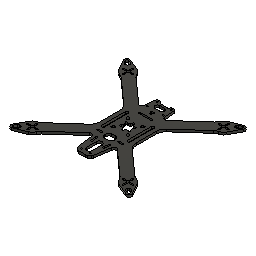
5inch test frame (Autodesk Fusion 360 design; units mm, degrees)
part number: 2026-08-20-13-27-36-607
Autodesk Fusion 360 part; units mm, degrees
note: some values were not read from the file. Chosen so that the rebuilt part matches the saved one: which bodies a step acts on.
(part 1 of 3)
sketch "reference" plane through (0, 0, 0) normal (0, 0, 1) x (1, 0, 0)
  line L0 (100, -100) -> (-100, -100) construction
  line L1 (-100, -100) -> (-100, 100) construction
  line L2 (-100, 100) -> (100, 100) construction
  line L3 (100, 100) -> (100, -100) construction
  line L4 (100, -100) -> (-100, 100) construction
  line L5 (-100, -100) -> (100, 100) construction
  circle A0 centre (-100, 100) radius 67.31
  circle A1 centre (100, 100) radius 67.31
  circle A2 centre (-100, -100) radius 67.31
  circle A3 centre (100, -100) radius 67.31
  line L6 (-32.69, 100) -> (32.69, 100)
  dimension "d1" = 134.62
  dimension "d2" = 134.62
  dimension "d3" = 134.62
  dimension "d4" = 134.62
  dimension "d5" = 200
  dimension "d7" = 200
  dimension "d8" = 65.38
  constraint horizontal L0
  constraint perpendicular L0 L1
  constraint parallel L0 L2
  constraint parallel L1 L3
  constraint coincident L4 origin
  constraint coincident L5 origin
  constraint coincident L1.end L2.start
  constraint coincident L2.end L3.start
  constraint coincident L0.end L1.start
  constraint coincident L0.start L3.end
  constraint equal L2 L3
  constraint coincident A0 L6.start
  constraint coincident L2 L6.start
  constraint coincident L2 L6.end
  constraint coincident A1 L6.end
  measures "d1" diameter of A0
  measures "d2" diameter of A1
  measures "d3" diameter of A2
  measures "d4" diameter of A3
  measures "d5" distance of L1.end L2.end
  measures "d7" distance of L0.start L2.end
  measures "d8" distance of L6.start L6.end
sketch "Sketch2" plane through (0, 0, 0) normal (0, 0, 1) x (1, 0, 0)
  circle A0 centre (-100, 100) radius 67.31 construction
  circle A1 centre (100, 100) radius 67.31 construction
  circle A2 centre (100, -100) radius 67.31 construction
  circle A3 centre (-100, -100) radius 67.31 construction
  line L0 (15.25, -15.25) -> (-15.25, -15.25) construction
  line L1 (-15.25, -15.25) -> (-15.25, 15.25) construction
  line L2 (-15.25, 15.25) -> (15.25, 15.25) construction
  line L3 (15.25, 15.25) -> (15.25, -15.25) construction
  line L4 (15.25, -15.25) -> (-15.25, 15.25) construction
  line L5 (-15.25, -15.25) -> (15.25, 15.25) construction
  line L6 (15.5328, 17.7956) -> (12.7044, 14.9672)
  arc A4 (12.7044, 14.9672) -> (14.9672, 12.7044) centre (13.8358, 13.8358) ccw
  line L7 (14.9672, 12.7044) -> (17.7956, 15.5328)
  arc A5 (17.7956, 15.5328) -> (15.5328, 17.7956) centre (16.6642, 16.6642) ccw
  line L8 (16.6642, 16.6642) -> (13.8358, 13.8358) construction
  arc A6 (-14.9672, 12.7044) -> (-12.7044, 14.9672) centre (-13.8358, 13.8358) ccw
  line L9 (-12.7044, 14.9672) -> (-15.5328, 17.7956)
  arc A7 (-15.5328, 17.7956) -> (-17.7956, 15.5328) centre (-16.6642, 16.6642) ccw
  line L10 (-17.7956, 15.5328) -> (-14.9672, 12.7044)
  arc A8 (-12.7044, -14.9672) -> (-14.9672, -12.7044) centre (-13.8358, -13.8358) ccw
  line L11 (-14.9672, -12.7044) -> (-17.7956, -15.5328)
  arc A9 (-17.7956, -15.5328) -> (-15.5328, -17.7956) centre (-16.6642, -16.6642) ccw
  line L12 (-15.5328, -17.7956) -> (-12.7044, -14.9672)
  arc A10 (14.9672, -12.7044) -> (12.7044, -14.9672) centre (13.8358, -13.8358) ccw
  line L13 (12.7044, -14.9672) -> (15.5328, -17.7956)
  arc A11 (15.5328, -17.7956) -> (17.7956, -15.5328) centre (16.6642, -16.6642) ccw
  line L14 (17.7956, -15.5328) -> (14.9672, -12.7044)
  circle A12 centre (-100, 100) radius 14.5
  circle A13 centre (-100, 100) radius 8 construction
  line L15 (-100, 100) -> (0, 0) construction
  line L16 (-100, 100) -> (-100, 92) construction
  line L17 (-98.4, 90) -> (-98.4, 94)
  arc A14 (-98.4, 94) -> (-101.6, 94) centre (-100, 94) ccw
  line L18 (-101.6, 94) -> (-101.6, 90)
  arc A15 (-101.6, 90) -> (-98.4, 90) centre (-100, 90) ccw
  line L19 (-100, 90) -> (-100, 94) construction
  arc A16 (-94, 101.6) -> (-94, 98.4) centre (-94, 100) ccw
  line L20 (-94, 98.4) -> (-90, 98.4)
  line L21 (-90, 101.6) -> (-94, 101.6)
  arc A17 (-90, 98.4) -> (-90, 101.6) centre (-90, 100) ccw
  arc A18 (-101.6, 106) -> (-98.4, 106) centre (-100, 106) ccw
  line L22 (-98.4, 106) -> (-98.4, 110)
  line L23 (-101.6, 110) -> (-101.6, 106)
  arc A19 (-98.4, 110) -> (-101.6, 110) centre (-100, 110) ccw
  arc A20 (-106, 98.4) -> (-106, 101.6) centre (-106, 100) ccw
  line L24 (-106, 101.6) -> (-110, 101.6)
  line L25 (-110, 98.4) -> (-106, 98.4)
  arc A21 (-110, 101.6) -> (-110, 98.4) centre (-110, 100) ccw
  circle A22 centre (-100, 100) radius 3
  line L26 (22, -45) -> (-22, -45) construction
  line L27 (-22, -45) -> (-22, 45) construction
  line L28 (-22, 45) -> (22, 45) construction
  line L29 (22, 45) -> (22, -45) construction
  line L30 (22, -45) -> (-22, 45) construction
  line L31 (-22, -45) -> (22, 45) construction
  line L32 (-27, -45) -> (-27, 45) construction
  line L33 (-30, 25) -> (-30, -25)
  arc A23 (-30, -25) -> (-24, -25) centre (-27, -25) ccw
  line L34 (-24, -25) -> (-24, 25)
  arc A24 (-24, 25) -> (-30, 25) centre (-27, 25) ccw
  line L35 (-27, 25) -> (-27, -25) construction
  line L36 (0, 0) -> (0, -45) construction
  line L37 (30, 25) -> (30, -25)
  arc A25 (30, 25) -> (24, 25) centre (27, 25) ccw
  line L38 (24, -25) -> (24, 25)
  arc A26 (24, -25) -> (30, -25) centre (27, -25) ccw
  line L39 (38, -45.25) -> (-38, -45.25)
  line L40 (-38, -45.25) -> (-38, 45.25)
  line L41 (-38, 45.25) -> (38, 45.25)
  line L42 (38, 45.25) -> (38, -45.25)
  line L43 (38, -45.25) -> (-38, 45.25) construction
  line L44 (-38, -45.25) -> (38, 45.25) construction
  point P0 (15.25, 15.25)
  point P1 (-100, 92)
  point P2 (-27, 0)
  dimension "d9" = 30.5
  dimension "d10" = 30.5
  dimension "d11" = 2
  dimension "d12" = 3.2
  dimension "d14" = 360
  dimension "d15" = 29
  dimension "d16" = 16
  dimension "d17" = 2
  dimension "d18" = 3.2
  dimension "d20" = 360
  dimension "d21" = 6
  dimension "d22" = 44
  dimension "d23" = 90
  dimension "d24" = -5
  dimension "d26" = 6
  dimension "d27" = 50
  dimension "d28" = 8
  dimension "d29" = 30
  constraint horizontal L0
  constraint perpendicular L0 L1
  constraint parallel L0 L2
  constraint parallel L1 L3
  constraint coincident L4 L15.end
  constraint coincident L5 L15.end
  constraint coincident L15.end L36.start
  constraint tangent L6 A4
  constraint tangent A4 L7
  constraint parallel L6 L7
  constraint tangent L7 A5
  constraint tangent L6 A5
  constraint coincident L5 A4.centre
  constraint parallel L5 L8
  constraint coincident P0 L2.end
  constraint midpoint L8 P0
  constraint concentric A0 A12
  constraint concentric A0 A13
  constraint coincident A0.centre A12.centre
  constraint coincident A13 P1
  constraint vertical L16
  constraint tangent L17 A14
  constraint tangent A14 L18
  constraint parallel L17 L18
  constraint tangent L18 A15
  constraint tangent L17 A15
  constraint coincident L16 A14.centre
  constraint parallel L16 L19
  constraint coincident P1 L16.end
  constraint midpoint L19 P1
  constraint concentric A0 A22
  constraint horizontal L26
  constraint perpendicular L26 L27
  constraint parallel L26 L28
  constraint parallel L27 L29
  constraint coincident L30 L15.end
  constraint coincident L31 L15.end
  constraint tangent L33 A23
  constraint tangent A23 L34
  constraint parallel L33 L34
  constraint tangent L34 A24
  constraint tangent L33 A24
  constraint coincident L32 A23.centre
  constraint parallel L32 L35
  constraint midpoint L32 P2
  constraint midpoint L35 P2
  constraint horizontal L26.end L32.start
  constraint horizontal L27.end L32.end
  constraint midpoint L26 L36.end
  constraint symmetric L33.start L36 L37.start
  constraint symmetric L33.end L36 L37.end
  constraint symmetric A23.end L36 L38.start
  constraint symmetric L34.end L36 A25.end
  constraint symmetric A23 L36 A26
  constraint symmetric A24 L36 A25
  constraint horizontal L39
  constraint perpendicular L39 L40
  constraint parallel L39 L41
  constraint parallel L40 L42
  constraint coincident L43 L15.end
  constraint coincident L44 L15.end
  measures "d9" distance of L1.end P0
  measures "d10" distance of L0.end L1.end
  measures "d11" distance of A4.centre P0
  measures "d12" diameter of A4
  measures "d15" diameter of A12
  measures "d16" diameter of A13
  measures "d17" distance of A14.centre P1
  measures "d18" diameter of A14
  measures "d21" diameter of A22
  measures "d22" distance of L27.end L28.end
  measures "d23" distance of L26.end L27.end
  measures "d26" diameter of A23
  measures "d27" distance of A24.centre A23.centre
  measures "d28" distance of L33 L40
  measures "d29" distance of L2 L41
  measures "d88" diameter of L37.start
extrude "Extrude1" add sketch "Sketch2" along normal blind 5 makes body 1 at (-106.0764, 105.8208, 0) makes body 2 at (-8.3765, 39.2818, 0)
fillet "Fillet1" radius 6 4 edges at (-38, -45.25, 2.5) (38, -45.25, 2.5) (38, 45.25, 2.5) (-38, 45.25, 2.5) on bodies 2
sketch "Sketch3" plane through (0, 0, 0) normal (0, 0, 1) x (1, 0, 0)
  arc A0 (-32, 45.25) -> (-38, 39.25) centre (-32, 39.25) ccw
  line L0 (-38, 39.25) -> (-38, -39.25)
  arc A1 (-38, -39.25) -> (-32, -45.25) centre (-32, -39.25) ccw
  line L1 (-32, -45.25) -> (32, -45.25)
  arc A2 (32, -45.25) -> (38, -39.25) centre (32, -39.25) ccw
  line L2 (38, -39.25) -> (38, 39.25)
  arc A3 (38, 39.25) -> (32, 45.25) centre (32, 39.25) ccw
  line L3 (32, 45.25) -> (-32, 45.25)
  arc A4 (30, 25) -> (24, 25) centre (27, 25) ccw
  line L4 (30, 25) -> (30, -25)
  arc A5 (24, -25) -> (30, -25) centre (27, -25) ccw
  line L5 (24, -25) -> (24, 25)
  arc A6 (17.7956, 15.5328) -> (15.5328, 17.7956) centre (16.6642, 16.6642) ccw
  line L6 (17.7956, 15.5328) -> (14.9672, 12.7044)
  arc A7 (12.7044, 14.9672) -> (14.9672, 12.7044) centre (13.8358, 13.8358) ccw
  line L7 (12.7044, 14.9672) -> (15.5328, 17.7956)
  line L8 (-12.7044, -14.9672) -> (-15.5328, -17.7956)
  arc A8 (-17.7956, -15.5328) -> (-15.5328, -17.7956) centre (-16.6642, -16.6642) ccw
  line L9 (-17.7956, -15.5328) -> (-14.9672, -12.7044)
  arc A9 (-12.7044, -14.9672) -> (-14.9672, -12.7044) centre (-13.8358, -13.8358) ccw
  line L10 (-14.9672, 12.7044) -> (-17.7956, 15.5328)
  arc A10 (-15.5328, 17.7956) -> (-17.7956, 15.5328) centre (-16.6642, 16.6642) ccw
  line L11 (-15.5328, 17.7956) -> (-12.7044, 14.9672)
  arc A11 (-14.9672, 12.7044) -> (-12.7044, 14.9672) centre (-13.8358, 13.8358) ccw
  arc A12 (-24, 25) -> (-30, 25) centre (-27, 25) ccw
  line L12 (-24, 25) -> (-24, -25)
  arc A13 (-30, -25) -> (-24, -25) centre (-27, -25) ccw
  line L13 (-30, -25) -> (-30, 25)
  line L14 (14.9672, -12.7044) -> (17.7956, -15.5328)
  arc A14 (15.5328, -17.7956) -> (17.7956, -15.5328) centre (16.6642, -16.6642) ccw
  line L15 (15.5328, -17.7956) -> (12.7044, -14.9672)
  arc A15 (14.9672, -12.7044) -> (12.7044, -14.9672) centre (13.8358, -13.8358) ccw
  arc A16 (-98.4, 110) -> (-101.6, 110) centre (-100, 110) ccw
  line L16 (-98.4, 110) -> (-98.4, 106)
  arc A17 (-101.6, 106) -> (-98.4, 106) centre (-100, 106) ccw
  line L17 (-101.6, 106) -> (-101.6, 110)
  circle A18 centre (-100, 100) radius 3
  arc A19 (-90, 98.4) -> (-90, 101.6) centre (-90, 100) ccw
  line L18 (-90, 98.4) -> (-94, 98.4)
  arc A20 (-94, 101.6) -> (-94, 98.4) centre (-94, 100) ccw
  line L19 (-94, 101.6) -> (-90, 101.6)
  arc A21 (-110, 101.6) -> (-110, 98.4) centre (-110, 100) ccw
  line L20 (-110, 101.6) -> (-106, 101.6)
  arc A22 (-106, 98.4) -> (-106, 101.6) centre (-106, 100) ccw
  line L21 (-106, 98.4) -> (-110, 98.4)
  arc A23 (-101.6, 90) -> (-98.4, 90) centre (-100, 90) ccw
  line L22 (-101.6, 90) -> (-101.6, 94)
  arc A24 (-98.4, 94) -> (-101.6, 94) centre (-100, 94) ccw
  line L23 (-98.4, 94) -> (-98.4, 90)
  circle A25 centre (-100, 100) radius 14.5
  line L24 (-100, 100) -> (-32, 39.25) construction
  line L25 (-109.6604, 89.1867) -> (-38, 25.1666)
  line L26 (-90.3396, 110.8133) -> (-16.9519, 45.25)
  line L27 (-100, 100) -> (-126.101, 123.3182) construction
  line L28 (-126.101, 123.3182) -> (-118.2572, 109.9935)
  line L29 (-118.2572, 109.9935) -> (-111.1861, 109.9935)
  line L30 (-126.101, 123.3182) -> (-111.1861, 117.0646)
  line L31 (-111.1861, 117.0646) -> (-111.1861, 109.9935)
  line L32 (-111.1861, 117.0646) -> (-118.2572, 109.9935) construction
  line L33 (-132.067, 128.648) -> (-112.7409, 93.0776)
  line L34 (-132.067, 128.648) -> (-94.5518, 113.4375)
  line L35 (-132.067, 128.648) -> (-126.101, 123.3182) construction
  line L36 (-100.2834, 85.5028) -> (-38, 29.8599)
  line L37 (-85.6262, 101.9091) -> (-22.2053, 45.25)
  dimension "d36" = 135
  dimension "d37" = 35
  dimension "d38" = 10
  dimension "d39" = 20
  dimension "d40" = 8
  dimension "d41" = 3.5
  dimension "d42" = 3.5
  dimension "d43" = 22
  constraint coincident A18.centre A25.centre
  constraint coincident A0.centre L24.end
  constraint coincident A25 L25.start
  constraint coincident L0 L25.end
  constraint coincident A25 L26.start
  constraint coincident L3 L26.end
  constraint parallel L24 L26
  constraint parallel L24 L25
  constraint tangent A25 L26
  constraint tangent A25 L25
  constraint parallel L24 L27
  constraint coincident L27 L29.end
  constraint horizontal L29
  constraint perpendicular L29 L31
  constraint coincident A25 L33.end
  constraint tangent A25 L33
  constraint coincident A25 L34.end
  constraint tangent A25 L34
  constraint parallel L27 L35
  constraint coincident A25 L36.start
  constraint coincident L0 L36.end
  constraint parallel L25 L36
  constraint coincident A25 L37.start
  constraint coincident L3 L37.end
  constraint parallel L26 L37
  measures "d36" angle of L29 L32
  measures "d37" distance of A18.centre L27.end
  measures "d38" distance of L28.end L30.end
  measures "d39" distance of L27.end L29.end
  measures "d40" distance of L27.end L33.start
  measures "d41" distance of L25 L36
  measures "d42" distance of L26 L37
  measures "d43" distance of L36 L37
extrude "Extrude2" add sketch "Sketch3" along normal blind 5 separate body contours A25 L33 L34 makes body 3
extrude "Extrude3" add sketch "Sketch3" along normal blind 5 separate body contours A0 L0 L3 A25 L36 L37 makes body 4
mirror "Mirror1" about plane through (0, 0, 0) normal (0, 1, 0) of bodies 3 1 4 makes body 5 at (-106.0764, -105.8208, 0) makes body 6 at (-121.5028, -111.8776, 0) makes body 7 at (-58.0639, -51.5744, 0)
mirror "Mirror2" about plane through (0, 0, 0) normal (1, 0, 0) of bodies 3 1 4 7 5 6 makes body 8 at (106.0764, 105.8208, 0) makes body 9 at (121.5028, 111.8776, 0) makes body 10 at (58.0639, 51.5744, 0) makes body 11 at (106.0764, -105.8208, 0) makes body 12 at (121.5028, -111.8776, 0) makes body 13 at (58.0639, -51.5744, 0)
combine "Combine1" operation add target body 2 tool bodies 11 3 13 1 5 6 10 7 4 8 9 12
fillet "Fillet2" radius 18 8 edges at (-100.2834, 85.5028, 2.5) (-85.6262, 101.9091, 2.5) (85.6262, 101.9091, 2.5) (100.2834, 85.5028, 2.5) (85.6262, -101.9091, 2.5) (100.2834, -85.5028, 2.5) (-100.2834, -85.5028, 2.5) (-85.6262, -101.9091, 2.5) on bodies 2
fillet "Fillet3" radius 2.5 16 edges at (-126.101, -123.3182, 2.5) (-118.2572, -109.9935, 2.5) (-111.1861, -109.9935, 2.5) (-111.1861, -117.0646, 2.5) (-111.1861, 117.0646, 2.5) (-126.101, 123.3182, 2.5) (-118.2572, 109.9935, 2.5) (-111.1861, 109.9935, 2.5) (126.101, 123.3182, 2.5) (111.1861, 117.0646, 2.5) (111.1861, 109.9935, 2.5) (118.2572, 109.9935, 2.5) (111.1861, -109.9935, 2.5) (118.2572, -109.9935, 2.5) (126.101, -123.3182, 2.5) (111.1861, -117.0646, 2.5) on bodies 2
fillet "Fillet4" radius 5 4 edges at (-132.067, -128.648, 2.5) (-132.067, 128.648, 2.5) (132.067, 128.648, 2.5) (132.067, -128.648, 2.5) on bodies 2
fillet "Fillet5" radius 20 4 edges at (-38, 29.8599, 2.5) (-38, -29.8599, 2.5) (38, 29.8599, 2.5) (38, -29.8599, 2.5) on bodies 2
sketch "Sketch4" plane through (0, 0, 5) normal (0, 0, 1) x (-1, 0, 0)
  arc A0 (-119.1307, 123.403) -> (-125.4028, 116.3824) centre (-121.0094, 118.7694) ccw
  line L0 (-125.4028, 116.3824) -> (-112.7409, 93.0776)
  arc A1 (-112.7409, 93.0776) -> (-103.7386, 85.9903) centre (-100, 100) ccw
  arc A2 (-96.3875, 82.0222) -> (-103.7386, 85.9903) centre (-108.3797, 68.5989) ccw
  line L1 (-96.3875, 82.0222) -> (-44.6753, 35.8235)
  arc A3 (-38, 20.9087) -> (-44.6753, 35.8235) centre (-58, 20.9087) ccw
  line L2 (-38, 20.9087) -> (-38, -20.9087)
  arc A4 (-44.6753, -35.8235) -> (-38, -20.9087) centre (-58, -20.9087) ccw
  line L3 (-44.6753, -35.8235) -> (-96.3875, -82.0222)
  arc A5 (-103.7386, -85.9903) -> (-96.3875, -82.0222) centre (-108.3797, -68.5989) ccw
  arc A6 (-103.7386, -85.9903) -> (-112.7409, -93.0776) centre (-100, -100) ccw
  line L4 (-112.7409, -93.0776) -> (-125.4028, -116.3824)
  arc A7 (-125.4028, -116.3824) -> (-119.1307, -123.403) centre (-121.0094, -118.7694) ccw
  line L5 (-119.1307, -123.403) -> (-94.5518, -113.4375)
  arc A8 (-94.5518, -113.4375) -> (-86.4985, -105.2878) centre (-100, -100) ccw
  arc A9 (-81.7303, -98.4286) -> (-86.4985, -105.2878) centre (-69.7381, -111.852) ccw
  line L6 (-81.7303, -98.4286) -> (-22.2053, -45.25)
  line L7 (-22.2053, -45.25) -> (22.2053, -45.25)
  line L8 (22.2053, -45.25) -> (81.7303, -98.4286)
  arc A10 (86.4985, -105.2878) -> (81.7303, -98.4286) centre (69.7381, -111.852) ccw
  arc A11 (86.4985, -105.2878) -> (94.5518, -113.4375) centre (100, -100) ccw
  line L9 (94.5518, -113.4375) -> (119.1307, -123.403)
  arc A12 (119.1307, -123.403) -> (125.4028, -116.3824) centre (121.0094, -118.7694) ccw
  line L10 (125.4028, -116.3824) -> (112.7409, -93.0776)
  arc A13 (112.7409, -93.0776) -> (103.7386, -85.9903) centre (100, -100) ccw
  arc A14 (96.3875, -82.0222) -> (103.7386, -85.9903) centre (108.3797, -68.5989) ccw
  line L11 (96.3875, -82.0222) -> (44.6753, -35.8235)
  arc A15 (38, -20.9087) -> (44.6753, -35.8235) centre (58, -20.9087) ccw
  line L12 (38, -20.9087) -> (38, 20.9087)
  arc A16 (44.6753, 35.8235) -> (38, 20.9087) centre (58, 20.9087) ccw
  line L13 (44.6753, 35.8235) -> (96.3875, 82.0222)
  arc A17 (103.7386, 85.9903) -> (96.3875, 82.0222) centre (108.3797, 68.5989) ccw
  arc A18 (103.7386, 85.9903) -> (112.7409, 93.0776) centre (100, 100) ccw
  line L14 (112.7409, 93.0776) -> (125.4028, 116.3824)
  arc A19 (125.4028, 116.3824) -> (119.1307, 123.403) centre (121.0094, 118.7694) ccw
  line L15 (119.1307, 123.403) -> (94.5518, 113.4375)
  arc A20 (94.5518, 113.4375) -> (86.4985, 105.2878) centre (100, 100) ccw
  arc A21 (81.7303, 98.4286) -> (86.4985, 105.2878) centre (69.7381, 111.852) ccw
  line L16 (81.7303, 98.4286) -> (22.2053, 45.25)
  line L17 (22.2053, 45.25) -> (-22.2053, 45.25)
  line L18 (-22.2053, 45.25) -> (-81.7303, 98.4286)
  arc A22 (-86.4985, 105.2878) -> (-81.7303, 98.4286) centre (-69.7381, 111.852) ccw
  arc A23 (-86.4985, 105.2878) -> (-94.5518, 113.4375) centre (-100, 100) ccw
  line L19 (-94.5518, 113.4375) -> (-119.1307, 123.403)
  line L20 (-118.9823, 111.2253) -> (-122.285, 116.8358)
  arc A24 (-119.1639, 120.4095) -> (-122.285, 116.8358) centre (-120.1306, 118.104) ccw
  line L21 (-119.1639, 120.4095) -> (-112.7195, 117.7075)
  arc A25 (-111.1861, 115.4019) -> (-112.7195, 117.7075) centre (-113.6861, 115.4019) ccw
  line L22 (-111.1861, 115.4019) -> (-111.1861, 112.4935)
  arc A26 (-113.6861, 109.9935) -> (-111.1861, 112.4935) centre (-113.6861, 112.4935) ccw
  line L23 (-113.6861, 109.9935) -> (-116.8279, 109.9935)
  arc A27 (-118.9823, 111.2253) -> (-116.8279, 109.9935) centre (-116.8279, 112.4935) ccw
  line L24 (-116.8279, -109.9935) -> (-113.6861, -109.9935)
  arc A28 (-111.1861, -112.4935) -> (-113.6861, -109.9935) centre (-113.6861, -112.4935) ccw
  line L25 (-111.1861, -112.4935) -> (-111.1861, -115.4019)
  arc A29 (-112.7195, -117.7075) -> (-111.1861, -115.4019) centre (-113.6861, -115.4019) ccw
  line L26 (-112.7195, -117.7075) -> (-119.1639, -120.4095)
  arc A30 (-122.285, -116.8358) -> (-119.1639, -120.4095) centre (-120.1306, -118.104) ccw
  line L27 (-122.285, -116.8358) -> (-118.9823, -111.2253)
  arc A31 (-116.8279, -109.9935) -> (-118.9823, -111.2253) centre (-116.8279, -112.4935) ccw
  arc A32 (-98.4, -90) -> (-101.6, -90) centre (-100, -90) ccw
  line L28 (-98.4, -90) -> (-98.4, -94)
  arc A33 (-101.6, -94) -> (-98.4, -94) centre (-100, -94) ccw
  line L29 (-101.6, -94) -> (-101.6, -90)
  arc A34 (-110, -98.4) -> (-110, -101.6) centre (-110, -100) ccw
  line L30 (-110, -98.4) -> (-106, -98.4)
  arc A35 (-106, -101.6) -> (-106, -98.4) centre (-106, -100) ccw
  line L31 (-106, -101.6) -> (-110, -101.6)
  arc A36 (-90, -101.6) -> (-90, -98.4) centre (-90, -100) ccw
  line L32 (-90, -101.6) -> (-94, -101.6)
  arc A37 (-94, -98.4) -> (-94, -101.6) centre (-94, -100) ccw
  line L33 (-94, -98.4) -> (-90, -98.4)
  circle A38 centre (-100, -100) radius 3
  arc A39 (-101.6, -110) -> (-98.4, -110) centre (-100, -110) ccw
  line L34 (-101.6, -110) -> (-101.6, -106)
  arc A40 (-98.4, -106) -> (-101.6, -106) centre (-100, -106) ccw
  line L35 (-98.4, -106) -> (-98.4, -110)
  line L36 (118.9823, -111.2253) -> (122.285, -116.8358)
  arc A41 (119.1639, -120.4095) -> (122.285, -116.8358) centre (120.1306, -118.104) ccw
  line L37 (119.1639, -120.4095) -> (112.7195, -117.7075)
  arc A42 (111.1861, -115.4019) -> (112.7195, -117.7075) centre (113.6861, -115.4019) ccw
  line L38 (111.1861, -115.4019) -> (111.1861, -112.4935)
  arc A43 (113.6861, -109.9935) -> (111.1861, -112.4935) centre (113.6861, -112.4935) ccw
  line L39 (113.6861, -109.9935) -> (116.8279, -109.9935)
  arc A44 (118.9823, -111.2253) -> (116.8279, -109.9935) centre (116.8279, -112.4935) ccw
  arc A45 (98.4, -110) -> (101.6, -110) centre (100, -110) ccw
  line L40 (98.4, -110) -> (98.4, -106)
  arc A46 (101.6, -106) -> (98.4, -106) centre (100, -106) ccw
  line L41 (101.6, -106) -> (101.6, -110)
  circle A47 centre (100, -100) radius 3
  arc A48 (90, -98.4) -> (90, -101.6) centre (90, -100) ccw
  line L42 (90, -98.4) -> (94, -98.4)
  arc A49 (94, -101.6) -> (94, -98.4) centre (94, -100) ccw
  line L43 (94, -101.6) -> (90, -101.6)
  arc A50 (110, -101.6) -> (110, -98.4) centre (110, -100) ccw
  line L44 (110, -101.6) -> (106, -101.6)
  arc A51 (106, -98.4) -> (106, -101.6) centre (106, -100) ccw
  line L45 (106, -98.4) -> (110, -98.4)
  arc A52 (101.6, -90) -> (98.4, -90) centre (100, -90) ccw
  line L46 (101.6, -90) -> (101.6, -94)
  arc A53 (98.4, -94) -> (101.6, -94) centre (100, -94) ccw
  line L47 (98.4, -94) -> (98.4, -90)
  arc A54 (98.4, 90) -> (101.6, 90) centre (100, 90) ccw
  line L48 (98.4, 90) -> (98.4, 94)
  arc A55 (101.6, 94) -> (98.4, 94) centre (100, 94) ccw
  line L49 (101.6, 94) -> (101.6, 90)
  arc A56 (110, 98.4) -> (110, 101.6) centre (110, 100) ccw
  line L50 (110, 98.4) -> (106, 98.4)
  arc A57 (106, 101.6) -> (106, 98.4) centre (106, 100) ccw
  line L51 (106, 101.6) -> (110, 101.6)
  arc A58 (90, 101.6) -> (90, 98.4) centre (90, 100) ccw
  line L52 (90, 101.6) -> (94, 101.6)
  arc A59 (94, 98.4) -> (94, 101.6) centre (94, 100) ccw
  line L53 (94, 98.4) -> (90, 98.4)
  circle A60 centre (100, 100) radius 3
  arc A61 (101.6, 110) -> (98.4, 110) centre (100, 110) ccw
  line L54 (101.6, 110) -> (101.6, 106)
  arc A62 (98.4, 106) -> (101.6, 106) centre (100, 106) ccw
  line L55 (98.4, 106) -> (98.4, 110)
  line L56 (112.7195, 117.7075) -> (119.1639, 120.4095)
  arc A63 (122.285, 116.8358) -> (119.1639, 120.4095) centre (120.1306, 118.104) ccw
  line L57 (122.285, 116.8358) -> (118.9823, 111.2253)
  arc A64 (116.8279, 109.9935) -> (118.9823, 111.2253) centre (116.8279, 112.4935) ccw
  line L58 (116.8279, 109.9935) -> (113.6861, 109.9935)
  arc A65 (111.1861, 112.4935) -> (113.6861, 109.9935) centre (113.6861, 112.4935) ccw
  line L59 (111.1861, 112.4935) -> (111.1861, 115.4019)
  arc A66 (112.7195, 117.7075) -> (111.1861, 115.4019) centre (113.6861, 115.4019) ccw
  line L60 (-14.9672, 12.7044) -> (-17.7956, 15.5328)
  arc A67 (-15.5328, 17.7956) -> (-17.7956, 15.5328) centre (-16.6642, 16.6642) ccw
  line L61 (-15.5328, 17.7956) -> (-12.7044, 14.9672)
  arc A68 (-14.9672, 12.7044) -> (-12.7044, 14.9672) centre (-13.8358, 13.8358) ccw
  arc A69 (24, -25) -> (30, -25) centre (27, -25) ccw
  line L62 (24, -25) -> (24, 25)
  arc A70 (30, 25) -> (24, 25) centre (27, 25) ccw
  line L63 (30, 25) -> (30, -25)
  line L64 (14.9672, -12.7044) -> (17.7956, -15.5328)
  arc A71 (15.5328, -17.7956) -> (17.7956, -15.5328) centre (16.6642, -16.6642) ccw
  line L65 (15.5328, -17.7956) -> (12.7044, -14.9672)
  arc A72 (14.9672, -12.7044) -> (12.7044, -14.9672) centre (13.8358, -13.8358) ccw
  line L66 (12.7044, 14.9672) -> (15.5328, 17.7956)
  arc A73 (17.7956, 15.5328) -> (15.5328, 17.7956) centre (16.6642, 16.6642) ccw
  line L67 (17.7956, 15.5328) -> (14.9672, 12.7044)
  arc A74 (12.7044, 14.9672) -> (14.9672, 12.7044) centre (13.8358, 13.8358) ccw
  arc A75 (-17.7956, -15.5328) -> (-15.5328, -17.7956) centre (-16.6642, -16.6642) ccw
  line L68 (-17.7956, -15.5328) -> (-14.9672, -12.7044)
  arc A76 (-12.7044, -14.9672) -> (-14.9672, -12.7044) centre (-13.8358, -13.8358) ccw
  line L69 (-12.7044, -14.9672) -> (-15.5328, -17.7956)
  arc A77 (-30, -25) -> (-24, -25) centre (-27, -25) ccw
  line L70 (-30, -25) -> (-30, 25)
  arc A78 (-24, 25) -> (-30, 25) centre (-27, 25) ccw
  line L71 (-24, 25) -> (-24, -25)
  arc A79 (-98.4, 110) -> (-101.6, 110) centre (-100, 110) ccw
  line L72 (-98.4, 110) -> (-98.4, 106)
  arc A80 (-101.6, 106) -> (-98.4, 106) centre (-100, 106) ccw
  line L73 (-101.6, 106) -> (-101.6, 110)
  circle A81 centre (-100, 100) radius 3
  arc A82 (-90, 98.4) -> (-90, 101.6) centre (-90, 100) ccw
  line L74 (-90, 98.4) -> (-94, 98.4)
  arc A83 (-94, 101.6) -> (-94, 98.4) centre (-94, 100) ccw
  line L75 (-94, 101.6) -> (-90, 101.6)
  arc A84 (-110, 101.6) -> (-110, 98.4) centre (-110, 100) ccw
  line L76 (-110, 101.6) -> (-106, 101.6)
  arc A85 (-106, 98.4) -> (-106, 101.6) centre (-106, 100) ccw
  line L77 (-106, 98.4) -> (-110, 98.4)
  arc A86 (-101.6, 90) -> (-98.4, 90) centre (-100, 90) ccw
  line L78 (-101.6, 90) -> (-101.6, 94)
  arc A87 (-98.4, 94) -> (-101.6, 94) centre (-100, 94) ccw
  line L79 (-98.4, 94) -> (-98.4, 90)
  line L80 (0, 45.25) -> (0, 95.25) construction
  line L81 (22.2053, 45.25) -> (15, 95.25)
  line L82 (15, 95.25) -> (0, 95.25)
  line L83 (-22.2053, 45.25) -> (-15, 95.25)
  line L84 (-15, 95.25) -> (0, 95.25)
  line L85 (22.2053, -45.25) -> (19.1432, -80.25)
  line L86 (19.1432, -80.25) -> (10, -79.4501)
  line L87 (10, -79.4501) -> (10, -75.25)
  line L88 (10, -75.25) -> (0, -75.25)
  line L89 (0, -75.25) -> (0, -45.25) construction
  line L90 (-22.2053, -45.25) -> (-19.1432, -80.25)
  line L91 (-19.1432, -80.25) -> (-10, -79.4501)
  line L92 (-10, -79.4501) -> (-10, -75.25)
  line L93 (-10, -75.25) -> (0, -75.25)
  dimension "d60" = 50
  dimension "d61" = 15
  dimension "d62" = 85
  dimension "d63" = 10
  dimension "d64" = 35
  dimension "d65" = 30
  constraint midpoint L17 L80.start
  constraint perpendicular L17 L80
  constraint coincident L16.end L17.start
  constraint perpendicular L80 L82
  constraint symmetric L82.end L80 L84.end
  constraint symmetric L80 L16.end L17.end
  constraint symmetric L80 L81.end L83.end
  constraint coincident L7.end L8.start
  constraint perpendicular L85 L86
  constraint perpendicular L87 L88
  constraint midpoint L7 L89.end
  constraint vertical L89
  constraint vertical L87
  constraint symmetric L7.end L89 L6.end
  constraint symmetric L85.end L89 L90.end
  constraint symmetric L86.end L89 L91.end
  constraint symmetric L87.end L89 L92.end
  constraint symmetric L88.end L89 L93.end
  measures "d60" distance of L80.start L80.end
  measures "d61" distance of L80.end L81.end
  measures "d62" angle of L7 L85
  measures "d63" distance of L87.end L88.end
  measures "d64" vertical distance of L7.end L85.end
  measures "d65" distance of L88.end L89.end
extrude "Extrude4" add sketch "Sketch4" against normal blind 5 contours L17 L81 L82 L83 L84 | L7 L85 L86 L87 L88 L90 L91 L92 L93 bodies 2
fillet "Fillet6" radius 5 4 edges at (-22.2053, -45.25, 2.5) (22.2053, -45.25, 2.5) (-22.2053, 45.25, 2.5) (22.2053, 45.25, 2.5) on bodies 2
chamfer "Chamfer1" distance 6 angle 45 2 edges at (-15, -95.25, 2.5) (15, -95.25, 2.5) on bodies 2
fillet "Fillet7" radius 5 4 edges at (-15.8558, -89.3113, 2.5) (-9, -95.25, 2.5) (9, -95.25, 2.5) (15.8558, -89.3113, 2.5) on bodies 2
fillet "Fillet8" radius 2.5 6 edges at (19.1432, 80.25, 2.5) (10, 79.4501, 2.5) (-10, 79.4501, 2.5) (-19.1432, 80.25, 2.5) (-10, 75.25, 2.5) (10, 75.25, 2.5) on bodies 2
sketch "Sketch5" plane through (0, 0, 5) normal (0, 0, 1) x (-1, 0, 0)
  arc A0 (16.6527, -80.0321) -> (19.3611, -77.7595) centre (16.8706, -77.5416) ccw
  line L0 (19.3611, -77.7595) -> (21.3355, -55.1918)
  arc A1 (29.6477, -51.8989) -> (21.3355, -55.1918) centre (26.3165, -55.6276) ccw
  line L1 (29.6477, -51.8989) -> (81.7303, -98.4286)
  arc A2 (86.4985, -105.2878) -> (81.7303, -98.4286) centre (69.7381, -111.852) ccw
  arc A3 (86.4985, -105.2878) -> (94.5518, -113.4375) centre (100, -100) ccw
  line L2 (94.5518, -113.4375) -> (119.1307, -123.403)
  arc A4 (119.1307, -123.403) -> (125.4028, -116.3824) centre (121.0094, -118.7694) ccw
  line L3 (125.4028, -116.3824) -> (112.7409, -93.0776)
  arc A5 (112.7409, -93.0776) -> (103.7386, -85.9903) centre (100, -100) ccw
  arc A6 (96.3875, -82.0222) -> (103.7386, -85.9903) centre (108.3797, -68.5989) ccw
  line L4 (96.3875, -82.0222) -> (44.6753, -35.8235)
  arc A7 (38, -20.9087) -> (44.6753, -35.8235) centre (58, -20.9087) ccw
  line L5 (38, -20.9087) -> (38, 20.9087)
  arc A8 (44.6753, 35.8235) -> (38, 20.9087) centre (58, 20.9087) ccw
  line L6 (44.6753, 35.8235) -> (96.3875, 82.0222)
  arc A9 (103.7386, 85.9903) -> (96.3875, 82.0222) centre (108.3797, 68.5989) ccw
  arc A10 (103.7386, 85.9903) -> (112.7409, 93.0776) centre (100, 100) ccw
  line L7 (112.7409, 93.0776) -> (125.4028, 116.3824)
  arc A11 (125.4028, 116.3824) -> (119.1307, 123.403) centre (121.0094, 118.7694) ccw
  line L8 (119.1307, 123.403) -> (94.5518, 113.4375)
  arc A12 (94.5518, 113.4375) -> (86.4985, 105.2878) centre (100, 100) ccw
  arc A13 (81.7303, 98.4286) -> (86.4985, 105.2878) centre (69.7381, 111.852) ccw
  line L9 (81.7303, 98.4286) -> (29.156, 51.4596)
  arc A14 (20.8759, 54.4751) -> (29.156, 51.4596) centre (25.8248, 55.1883) ccw
  line L10 (20.8759, 54.4751) -> (16.1217, 87.466)
  arc A15 (16.1217, 87.466) -> (14.4465, 90.5321) centre (11.1729, 86.7528) ccw
  line L11 (14.4465, 90.5321) -> (10.4093, 94.0293)
  arc A16 (10.4093, 94.0293) -> (7.1356, 95.25) centre (7.1356, 90.25) ccw
  line L12 (7.1356, 95.25) -> (-7.1356, 95.25)
  arc A17 (-7.1356, 95.25) -> (-10.4093, 94.0293) centre (-7.1356, 90.25) ccw
  line L13 (-10.4093, 94.0293) -> (-14.4465, 90.5321)
  arc A18 (-14.4465, 90.5321) -> (-16.1217, 87.466) centre (-11.1729, 86.7528) ccw
  line L14 (-16.1217, 87.466) -> (-20.8759, 54.4751)
  arc A19 (-29.156, 51.4596) -> (-20.8759, 54.4751) centre (-25.8248, 55.1883) ccw
  line L15 (-29.156, 51.4596) -> (-81.7303, 98.4286)
  arc A20 (-86.4985, 105.2878) -> (-81.7303, 98.4286) centre (-69.7381, 111.852) ccw
  arc A21 (-86.4985, 105.2878) -> (-94.5518, 113.4375) centre (-100, 100) ccw
  line L16 (-94.5518, 113.4375) -> (-119.1307, 123.403)
  arc A22 (-119.1307, 123.403) -> (-125.4028, 116.3824) centre (-121.0094, 118.7694) ccw
  line L17 (-125.4028, 116.3824) -> (-112.7409, 93.0776)
  arc A23 (-112.7409, 93.0776) -> (-103.7386, 85.9903) centre (-100, 100) ccw
  arc A24 (-96.3875, 82.0222) -> (-103.7386, 85.9903) centre (-108.3797, 68.5989) ccw
  line L18 (-96.3875, 82.0222) -> (-44.6753, 35.8235)
  arc A25 (-38, 20.9087) -> (-44.6753, 35.8235) centre (-58, 20.9087) ccw
  line L19 (-38, 20.9087) -> (-38, -20.9087)
  arc A26 (-44.6753, -35.8235) -> (-38, -20.9087) centre (-58, -20.9087) ccw
  line L20 (-44.6753, -35.8235) -> (-96.3875, -82.0222)
  arc A27 (-103.7386, -85.9903) -> (-96.3875, -82.0222) centre (-108.3797, -68.5989) ccw
  arc A28 (-103.7386, -85.9903) -> (-112.7409, -93.0776) centre (-100, -100) ccw
  line L21 (-112.7409, -93.0776) -> (-125.4028, -116.3824)
  arc A29 (-125.4028, -116.3824) -> (-119.1307, -123.403) centre (-121.0094, -118.7694) ccw
  line L22 (-119.1307, -123.403) -> (-94.5518, -113.4375)
  arc A30 (-94.5518, -113.4375) -> (-86.4985, -105.2878) centre (-100, -100) ccw
  arc A31 (-81.7303, -98.4286) -> (-86.4985, -105.2878) centre (-69.7381, -111.852) ccw
  line L23 (-81.7303, -98.4286) -> (-29.6477, -51.8989)
  arc A32 (-21.3355, -55.1918) -> (-29.6477, -51.8989) centre (-26.3165, -55.6276) ccw
  line L24 (-21.3355, -55.1918) -> (-19.3611, -77.7595)
  arc A33 (-19.3611, -77.7595) -> (-16.6527, -80.0321) centre (-16.8706, -77.5416) ccw
  line L25 (-16.6527, -80.0321) -> (-12.2821, -79.6497)
  arc A34 (-12.2821, -79.6497) -> (-10.0175, -77.4546) centre (-12.5, -77.1592) ccw
  arc A35 (-7.535, -75.25) -> (-10.0175, -77.4546) centre (-7.535, -77.75) ccw
  line L26 (-7.535, -75.25) -> (7.535, -75.25)
  arc A36 (10.0175, -77.4546) -> (7.535, -75.25) centre (7.535, -77.75) ccw
  arc A37 (10.0175, -77.4546) -> (12.2821, -79.6497) centre (12.5, -77.1592) ccw
  line L27 (12.2821, -79.6497) -> (16.6527, -80.0321)
  line L28 (-118.9823, 111.2253) -> (-122.285, 116.8358)
  arc A38 (-119.1639, 120.4095) -> (-122.285, 116.8358) centre (-120.1306, 118.104) ccw
  line L29 (-119.1639, 120.4095) -> (-112.7195, 117.7075)
  arc A39 (-111.1861, 115.4019) -> (-112.7195, 117.7075) centre (-113.6861, 115.4019) ccw
  line L30 (-111.1861, 115.4019) -> (-111.1861, 112.4935)
  arc A40 (-113.6861, 109.9935) -> (-111.1861, 112.4935) centre (-113.6861, 112.4935) ccw
  line L31 (-113.6861, 109.9935) -> (-116.8279, 109.9935)
  arc A41 (-118.9823, 111.2253) -> (-116.8279, 109.9935) centre (-116.8279, 112.4935) ccw
  line L32 (-116.8279, -109.9935) -> (-113.6861, -109.9935)
  arc A42 (-111.1861, -112.4935) -> (-113.6861, -109.9935) centre (-113.6861, -112.4935) ccw
  line L33 (-111.1861, -112.4935) -> (-111.1861, -115.4019)
  arc A43 (-112.7195, -117.7075) -> (-111.1861, -115.4019) centre (-113.6861, -115.4019) ccw
  line L34 (-112.7195, -117.7075) -> (-119.1639, -120.4095)
  arc A44 (-122.285, -116.8358) -> (-119.1639, -120.4095) centre (-120.1306, -118.104) ccw
  line L35 (-122.285, -116.8358) -> (-118.9823, -111.2253)
  arc A45 (-116.8279, -109.9935) -> (-118.9823, -111.2253) centre (-116.8279, -112.4935) ccw
  arc A46 (-98.4, -90) -> (-101.6, -90) centre (-100, -90) ccw
  line L36 (-98.4, -90) -> (-98.4, -94)
  arc A47 (-101.6, -94) -> (-98.4, -94) centre (-100, -94) ccw
  line L37 (-101.6, -94) -> (-101.6, -90)
  arc A48 (-110, -98.4) -> (-110, -101.6) centre (-110, -100) ccw
  line L38 (-110, -98.4) -> (-106, -98.4)
  arc A49 (-106, -101.6) -> (-106, -98.4) centre (-106, -100) ccw
  line L39 (-106, -101.6) -> (-110, -101.6)
  arc A50 (-90, -101.6) -> (-90, -98.4) centre (-90, -100) ccw
  line L40 (-90, -101.6) -> (-94, -101.6)
  arc A51 (-94, -98.4) -> (-94, -101.6) centre (-94, -100) ccw
  line L41 (-94, -98.4) -> (-90, -98.4)
  circle A52 centre (-100, -100) radius 3
  arc A53 (-101.6, -110) -> (-98.4, -110) centre (-100, -110) ccw
  line L42 (-101.6, -110) -> (-101.6, -106)
  arc A54 (-98.4, -106) -> (-101.6, -106) centre (-100, -106) ccw
  line L43 (-98.4, -106) -> (-98.4, -110)
  line L44 (118.9823, -111.2253) -> (122.285, -116.8358)
  arc A55 (119.1639, -120.4095) -> (122.285, -116.8358) centre (120.1306, -118.104) ccw
  line L45 (119.1639, -120.4095) -> (112.7195, -117.7075)
  arc A56 (111.1861, -115.4019) -> (112.7195, -117.7075) centre (113.6861, -115.4019) ccw
  line L46 (111.1861, -115.4019) -> (111.1861, -112.4935)
  arc A57 (113.6861, -109.9935) -> (111.1861, -112.4935) centre (113.6861, -112.4935) ccw
  line L47 (113.6861, -109.9935) -> (116.8279, -109.9935)
  arc A58 (118.9823, -111.2253) -> (116.8279, -109.9935) centre (116.8279, -112.4935) ccw
  arc A59 (98.4, -110) -> (101.6, -110) centre (100, -110) ccw
  line L48 (98.4, -110) -> (98.4, -106)
  arc A60 (101.6, -106) -> (98.4, -106) centre (100, -106) ccw
  line L49 (101.6, -106) -> (101.6, -110)
  circle A61 centre (100, -100) radius 3
  arc A62 (90, -98.4) -> (90, -101.6) centre (90, -100) ccw
  line L50 (90, -98.4) -> (94, -98.4)
  arc A63 (94, -101.6) -> (94, -98.4) centre (94, -100) ccw
  line L51 (94, -101.6) -> (90, -101.6)
  arc A64 (110, -101.6) -> (110, -98.4) centre (110, -100) ccw
  line L52 (110, -101.6) -> (106, -101.6)
  arc A65 (106, -98.4) -> (106, -101.6) centre (106, -100) ccw
  line L53 (106, -98.4) -> (110, -98.4)
  arc A66 (101.6, -90) -> (98.4, -90) centre (100, -90) ccw
  line L54 (101.6, -90) -> (101.6, -94)
  arc A67 (98.4, -94) -> (101.6, -94) centre (100, -94) ccw
  line L55 (98.4, -94) -> (98.4, -90)
  arc A68 (98.4, 90) -> (101.6, 90) centre (100, 90) ccw
  line L56 (98.4, 90) -> (98.4, 94)
  arc A69 (101.6, 94) -> (98.4, 94) centre (100, 94) ccw
  line L57 (101.6, 94) -> (101.6, 90)
  arc A70 (110, 98.4) -> (110, 101.6) centre (110, 100) ccw
  line L58 (110, 98.4) -> (106, 98.4)
  arc A71 (106, 101.6) -> (106, 98.4) centre (106, 100) ccw
  line L59 (106, 101.6) -> (110, 101.6)
  arc A72 (90, 101.6) -> (90, 98.4) centre (90, 100) ccw
  line L60 (90, 101.6) -> (94, 101.6)
  arc A73 (94, 98.4) -> (94, 101.6) centre (94, 100) ccw
  line L61 (94, 98.4) -> (90, 98.4)
  circle A74 centre (100, 100) radius 3
  arc A75 (101.6, 110) -> (98.4, 110) centre (100, 110) ccw
  line L62 (101.6, 110) -> (101.6, 106)
  arc A76 (98.4, 106) -> (101.6, 106) centre (100, 106) ccw
  line L63 (98.4, 106) -> (98.4, 110)
  line L64 (112.7195, 117.7075) -> (119.1639, 120.4095)
  arc A77 (122.285, 116.8358) -> (119.1639, 120.4095) centre (120.1306, 118.104) ccw
  line L65 (122.285, 116.8358) -> (118.9823, 111.2253)
  arc A78 (116.8279, 109.9935) -> (118.9823, 111.2253) centre (116.8279, 112.4935) ccw
  line L66 (116.8279, 109.9935) -> (113.6861, 109.9935)
  arc A79 (111.1861, 112.4935) -> (113.6861, 109.9935) centre (113.6861, 112.4935) ccw
  line L67 (111.1861, 112.4935) -> (111.1861, 115.4019)
  arc A80 (112.7195, 117.7075) -> (111.1861, 115.4019) centre (113.6861, 115.4019) ccw
  line L68 (-14.9672, 12.7044) -> (-17.7956, 15.5328)
  arc A81 (-15.5328, 17.7956) -> (-17.7956, 15.5328) centre (-16.6642, 16.6642) ccw
  line L69 (-15.5328, 17.7956) -> (-12.7044, 14.9672)
  arc A82 (-14.9672, 12.7044) -> (-12.7044, 14.9672) centre (-13.8358, 13.8358) ccw
  arc A83 (24, -25) -> (30, -25) centre (27, -25) ccw
  line L70 (24, -25) -> (24, 25)
  arc A84 (30, 25) -> (24, 25) centre (27, 25) ccw
  line L71 (30, 25) -> (30, -25)
  line L72 (14.9672, -12.7044) -> (17.7956, -15.5328)
  arc A85 (15.5328, -17.7956) -> (17.7956, -15.5328) centre (16.6642, -16.6642) ccw
  line L73 (15.5328, -17.7956) -> (12.7044, -14.9672)
  arc A86 (14.9672, -12.7044) -> (12.7044, -14.9672) centre (13.8358, -13.8358) ccw
  line L74 (12.7044, 14.9672) -> (15.5328, 17.7956)
  arc A87 (17.7956, 15.5328) -> (15.5328, 17.7956) centre (16.6642, 16.6642) ccw
  line L75 (17.7956, 15.5328) -> (14.9672, 12.7044)
  arc A88 (12.7044, 14.9672) -> (14.9672, 12.7044) centre (13.8358, 13.8358) ccw
  arc A89 (-17.7956, -15.5328) -> (-15.5328, -17.7956) centre (-16.6642, -16.6642) ccw
  line L76 (-17.7956, -15.5328) -> (-14.9672, -12.7044)
  arc A90 (-12.7044, -14.9672) -> (-14.9672, -12.7044) centre (-13.8358, -13.8358) ccw
  line L77 (-12.7044, -14.9672) -> (-15.5328, -17.7956)
  arc A91 (-30, -25) -> (-24, -25) centre (-27, -25) ccw
  line L78 (-30, -25) -> (-30, 25)
  arc A92 (-24, 25) -> (-30, 25) centre (-27, 25) ccw
  line L79 (-24, 25) -> (-24, -25)
  arc A93 (-98.4, 110) -> (-101.6, 110) centre (-100, 110) ccw
  line L80 (-98.4, 110) -> (-98.4, 106)
  arc A94 (-101.6, 106) -> (-98.4, 106) centre (-100, 106) ccw
  line L81 (-101.6, 106) -> (-101.6, 110)
  circle A95 centre (-100, 100) radius 3
  arc A96 (-90, 98.4) -> (-90, 101.6) centre (-90, 100) ccw
  line L82 (-90, 98.4) -> (-94, 98.4)
  arc A97 (-94, 101.6) -> (-94, 98.4) centre (-94, 100) ccw
  line L83 (-94, 101.6) -> (-90, 101.6)
  arc A98 (-110, 101.6) -> (-110, 98.4) centre (-110, 100) ccw
  line L84 (-110, 101.6) -> (-106, 101.6)
  arc A99 (-106, 98.4) -> (-106, 101.6) centre (-106, 100) ccw
  line L85 (-106, 98.4) -> (-110, 98.4)
  arc A100 (-101.6, 90) -> (-98.4, 90) centre (-100, 90) ccw
  line L86 (-101.6, 90) -> (-101.6, 94)
  arc A101 (-98.4, 94) -> (-101.6, 94) centre (-100, 94) ccw
  line L87 (-98.4, 94) -> (-98.4, 90)
  line L88 (16.8706, -77.5416) -> (12.5, -77.1592) construction
  line L89 (-12.5, -77.1592) -> (-16.8706, -77.5416) construction
  line L90 (0, 0) -> (0, 95.25) construction
  line L91 (14.6853, -77.3504) -> (16.6189, -55.25) construction
  line L92 (-14.6853, -77.3504) -> (-16.6189, -55.25) construction
  line L93 (16.6189, -55.25) -> (-16.6189, -55.25) construction
  circle A102 centre (14.8248, -75.7565) radius 1.6
  circle A103 centre (-14.8248, -75.7565) radius 1.6
  circle A104 centre (16.4789, -56.85) radius 1.6
  circle A105 centre (-16.4789, -56.85) radius 1.6
  line L94 (6, 60.25) -> (6, 80.25)
  arc A106 (6, 80.25) -> (-6, 80.25) centre (0, 80.25) ccw
  line L95 (-6, 80.25) -> (-6, 60.25)
  arc A107 (-6, 60.25) -> (6, 60.25) centre (0, 60.25) ccw
  line L96 (0, 60.25) -> (0, 80.25) construction
  line L97 (27, -25) -> (-27, -25) construction
  line L98 (27, 25) -> (-27, 25) construction
  line L99 (-10, 45) -> (10, 45)
  line L100 (10, 45) -> (10, 30)
  line L101 (10, 30) -> (-10, 30)
  line L102 (-10, 30) -> (-10, 45)
  line L103 (-10, 45) -> (10, 30) construction
  line L104 (10, 45) -> (-10, 30) construction
  line L105 (46.1228, -37) -> (-46.1228, -37) construction
  line L106 (46.1228, 37) -> (-46.1228, 37) construction
  line L107 (12.5, -35.4) -> (-12.5, -35.4)
  arc A108 (-12.5, -35.4) -> (-12.5, -38.6) centre (-12.5, -37) ccw
  line L108 (-12.5, -38.6) -> (12.5, -38.6)
  arc A109 (12.5, -38.6) -> (12.5, -35.4) centre (12.5, -37) ccw
  line L109 (12.5, -37) -> (-12.5, -37) construction
  line L110 (27, 25) -> (27, 37) construction
  line L111 (-18, 38.6) -> (-26, 38.6)
  arc A110 (-26, 38.6) -> (-26, 35.4) centre (-26, 37) ccw
  line L112 (-26, 35.4) -> (-18, 35.4)
  arc A111 (-18, 35.4) -> (-18, 38.6) centre (-18, 37) ccw
  line L113 (-18, 37) -> (-26, 37) construction
  arc A112 (18, 38.6) -> (18, 35.4) centre (18, 37) ccw
  line L114 (26, 35.4) -> (18, 35.4)
  line L115 (18, 38.6) -> (26, 38.6)
  arc A113 (26, 35.4) -> (26, 38.6) centre (26, 37) ccw
  line L116 (15.6521, -66.3002) -> (-15.6521, -66.3002) construction
  line L117 (5, -61.3002) -> (-5, -61.3002)
  arc A114 (-5, -61.3002) -> (-5, -71.3002) centre (-5, -66.3002) ccw
  line L118 (-5, -71.3002) -> (5, -71.3002)
  arc A115 (5, -71.3002) -> (5, -61.3002) centre (5, -66.3002) ccw
  line L119 (5, -66.3002) -> (-5, -66.3002) construction
  point P0 (0, 70.25)
  point P1 (0, 37.5)
  point P2 (0, -37)
  point P3 (-22, 37)
  point P4 (0, -66.3002)
  dimension "d75" = 20
  dimension "d76" = 3.2
  dimension "d77" = 3.2
  dimension "d78" = 3.2
  dimension "d79" = 3.2
  dimension "d80" = 12
  dimension "d81" = 20
  dimension "d82" = 15
  dimension "d83" = 20
  dimension "d84" = 15
  dimension "d85" = 5
  dimension "d86" = 12
  dimension "d87" = 12
  dimension "d88" = 3.2
  dimension "d89" = 25
  dimension "d90" = 3.2
  dimension "d91" = 8
  dimension "d92" = 8
  dimension "d93" = 10
  dimension "d94" = 10
  constraint coincident A0.centre L88.start
  constraint coincident A37.centre L88.end
  constraint coincident A34.centre L89.start
  constraint coincident A33.centre L89.end
  constraint coincident L90.start origin
  constraint midpoint L12 L90.end
  constraint midpoint L88 L91.start
  constraint midpoint L89 L92.start
  constraint horizontal L93
  constraint coincident L91 A102.centre
  constraint coincident L92 A103.centre
  constraint tangent L88 A102
  constraint tangent L89 A103
  constraint coincident L91 A104.centre
  constraint coincident L92 A105.centre
  constraint tangent L93 A104
  constraint tangent L93 A105
  constraint parallel L0 L91
  constraint parallel L24 L92
  constraint tangent L94 A106
  constraint tangent A106 L95
  constraint parallel L94 L95
  constraint tangent L95 A107
  constraint tangent L94 A107
  constraint parallel L90 L96
  constraint coincident L90 P0
  constraint midpoint L96 P0
  constraint coincident A83.centre L97.start
  constraint coincident A91.centre L97.end
  constraint coincident A84.centre L98.start
  constraint coincident A92.centre L98.end
  constraint horizontal L99
  constraint perpendicular L99 L100
  constraint parallel L99 L101
  constraint parallel L100 L102
  constraint coincident L103 P1
  constraint coincident L104 P1
  constraint coincident L90 P1
  constraint coincident A7 L105.start
  constraint coincident A26 L105.end
  constraint horizontal L105
  constraint coincident A8 L106.start
  constraint coincident A25 L106.end
  constraint perpendicular L90 L106
  constraint tangent L107 A108
  constraint tangent A108 L108
  constraint parallel L107 L108
  constraint tangent L108 A109
  constraint tangent L107 A109
  constraint coincident L105 A108.centre
  constraint perpendicular L71 L109
  constraint midpoint L105 P2
  constraint midpoint L109 P2
  constraint coincident L106 L110.end
  constraint perpendicular L106 L110
  constraint tangent L111 A110
  constraint tangent A110 L112
  constraint parallel L111 L112
  constraint tangent L112 A111
  constraint tangent L111 A111
  constraint coincident L106 A110.centre
  constraint midpoint L113 P3
  constraint coincident L106 P3
  constraint symmetric L90 L111.start A112.start
  constraint symmetric L90 L111.end L115.end
  constraint symmetric L90 A110.end L114.start
  constraint symmetric L90 L112.end A112.end
  constraint symmetric L90 A110 A113
  constraint symmetric L90 A111 A112
  constraint midpoint L91 L116.start
  constraint midpoint L92 L116.end
  constraint tangent L117 A114
  constraint tangent A114 L118
  constraint parallel L117 L118
  constraint tangent L118 A115
  constraint tangent L117 A115
  constraint coincident L116 A114.centre
  constraint parallel L116 L119
  constraint midpoint L116 P4
  constraint midpoint L119 P4
  measures "d75" distance of L26 L93
  measures "d76" diameter of A102
  measures "d77" diameter of A103
  measures "d78" diameter of A104
  measures "d79" diameter of A105
  measures "d80" diameter of A106
  measures "d81" distance of A107.centre A106.centre
  measures "d82" distance of L12 A106.centre
  measures "d83" distance of L100.end L101.end
  measures "d84" distance of L99.end L100.end
  measures "d85" distance of L98 L101
  measures "d86" distance of L98 L106
  measures "d87" distance of L97 L105
  measures "d88" diameter of A108
  measures "d89" distance of A109.centre A108.centre
  measures "d90" diameter of A110
  measures "d91" distance of A111.centre A110.centre
  measures "d92" distance of L102 A111.centre
  measures "d93" diameter of A114
  measures "d94" distance of A115.centre A114.centre
extrude "Extrude5" cut sketch "Sketch5" against normal blind 5 contours A102 | A103 | A104 | A105 | L94 A106 L95 A107 | L99 L100 L101 L102 | L107 A108 L108 A109 | L111 A110 L112 A111 | A112 L114 L115 A113 | L117 A114 L118 A115 bodies 2
fillet "Fillet9" radius 6 4 edges at (-10, -30, 2.5) (-10, -45, 2.5) (10, -45, 2.5) (10, -30, 2.5) on bodies 2